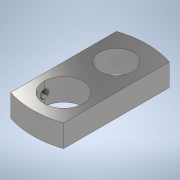
# Autodesk Inventor part: Part14
Saved by Autodesk Inventor 2020 (Build 240168000, 168)
## iProperties
Created: 2021-10-25
Part Number: Part14
Material: Steel, Mild
Document SubType Name: Modeling
Designer: simon.erikssonwestl
Density: 7.85 g/cm^3
Appearance: Semi-Polished
Author: simon.erikssonwestl
Autodesk Inventor part; units mm, degrees
ref_plane "YZ Plane" through (0, 0, 0) normal (1, 0, 0) x (0, 1, 0)
ref_plane "XZ Plane" through (0, 0, 0) normal (0, 1, 0) x (-1, 0, 0)
ref_plane "XY Plane" through (0, 0, 0) normal (0, 0, 1) x (1, 0, 0)
sketch "Sketch1" plane through (0, 0, 0) normal (0, 1, 0) x (-1, 0, 0)
  line L0 (4.75, 9.5) -> (-4.75, 9.5)
  line L1 (-4.75, 9.5) -> (-4.75, -9.5)
  line L2 (-4.75, -9.5) -> (4.75, -9.5)
  line L3 (4.75, -9.5) -> (4.75, 9.5)
  line L4 (4.75, 9.5) -> (-4.75, -9.5) construction
  line L5 (-4.75, 9.5) -> (4.75, -9.5) construction
  arc A0 (-4.75, -9.5) -> (4.75, -9.5) centre (0, 4.7281) ccw
  arc A1 (4.75, 9.5) -> (-4.75, 9.5) centre (0, -4.7281) ccw
  point P0 (0, 0)
  dimension "d0" = 9.5
  dimension "d1" = 19
  dimension "d2" = 15
  dimension "d3" = 15
  constraints: 12 end point, 4 point on circle, 2 centre point, 2 midpoint, 2 parallel, 1 horizontal, 1 perpendicular
  measures "d0" distance of L2.end L1.end
  measures "d1" distance of L1.end L0.end
  measures "d2" radius of A0
  measures "d3" radius of A1
extrude "Extrusion1" add sketch "Sketch1" along normal blind 4
sketch "Sketch2" plane through (0, 4, 0) normal (0, 1, 0) x (1, 0, 0)
  arc A0 (4.75, 9.5) -> (-4.75, 9.5) centre (0, -4.7281) ccw projected
  point P0 (0, 0)
  point P1 (0, 4.75)
  point P2 (0, -4.75)
  dimension "d6" = 4.75
  dimension "d7" = 9.5
  measures "d6" horizontal distance of point (0, 4.75) A0.end
  measures "d7" distance of point (0, 4.75) point (0, -4.75)
hole "Hole1" at (0, 4, -4.75) direction (0, -1, 0) diameter 6 end through all
hole "Hole2" at (0, 4, 4.75) at (0, 4, 4.7281) direction (0, -1, 0) diameter 7 end through all
sketch "Sketch3" plane through (-4.75, 0, -9.5) normal (-1, 0, 0) x (0, 0, 1)
  line L0 (19, 0) -> (19, 4) projected
  line L1 (0, 4) -> (19, 4) projected
  point P0 (9.5, 0)
  point P1 (14.25, 2)
  dimension "d22" = 4.75
  dimension "d23" = 2
  measures "d22" distance from line of L0 point (14.25, 2)
  measures "d23" distance from line of L1 point (14.25, 2)
hole "Hole3" at (-4.75, 2, 4.75) direction (1, 0, 0) diameter 1.5 depth 1.33 tip angle 118
body "Solid1"
